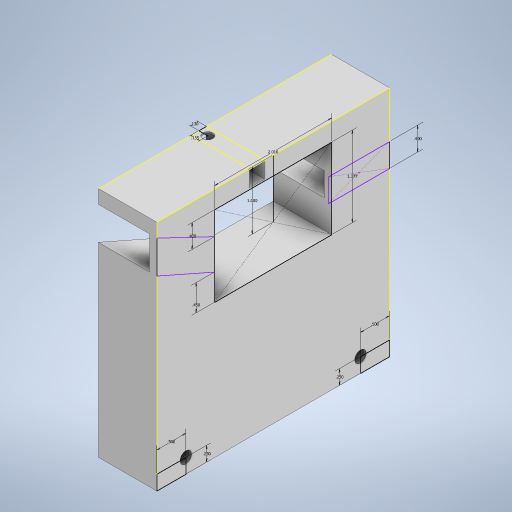
# Autodesk Inventor part: Al thermal core
Saved by Autodesk Inventor 2024.1 (Build 281209000, 209)
## iProperties
Created: 2024-08-21
Part Number: Al thermal core
Material: Generic
Document SubType Name: Modeling
Designer: pab2
Density: 1 g/cm^3
Appearance: Default
Author: pab2
Autodesk Inventor part; units mm, degrees
ref_plane "YZ Plane" through (0, 0, 0) normal (1, 0, 0) x (0, 1, 0)
ref_plane "XZ Plane" through (0, 0, 0) normal (0, 1, 0) x (-1, 0, 0)
ref_plane "XY Plane" through (0, 0, 0) normal (0, 0, 1) x (1, 0, 0)
sketch "Sketch1" plane through (0, 0, 0) normal (1, 0, 0) x (0, 1, 0)
  line L0 (0, 0) -> (101.6, 0)
  line L1 (101.6, 0) -> (101.6, -101.6)
  line L2 (101.6, -101.6) -> (0, -101.6)
  line L3 (0, -101.6) -> (0, 0)
  dimension "d0" = 101.6
  dimension "d1" = 101.6
  constraints: 8 end point, 2 parallel, 1 horizontal, 1 perpendicular
  measures "d0" distance of L1.end L2.end
  measures "d1" distance of L0.end L1.end
extrude "Extrusion1" add sketch "Sketch1" along normal blind 25.4
sketch "Sketch2" plane through (25.4, 0, 0) normal (1, 0, 0) x (0, 0, -1)
  line L0 (0, 101.6) -> (0, 0) projected
  line L1 (0, 0) -> (12.7, 0)
  line L2 (12.7, 0) -> (12.7, 6.35)
  line L3 (12.7, 6.35) -> (0, 6.35)
  line L4 (0, 6.35) -> (0, 0)
  line L5 (101.6, 0) -> (101.6, 101.6) projected
  line L6 (101.6, 0) -> (88.9, 0)
  line L7 (88.9, 0) -> (88.9, 6.35)
  line L8 (88.9, 6.35) -> (101.6, 6.35)
  line L9 (101.6, 6.35) -> (101.6, 0)
  line L10 (101.6, 101.6) -> (0, 101.6) projected
  line L11 (50.8, 101.6) -> (50.8, 76.2)
  line L12 (25.273, 58.7121) -> (76.327, 58.7121)
  line L13 (76.327, 58.7121) -> (76.327, 93.6879)
  line L14 (76.327, 93.6879) -> (25.273, 93.6879)
  line L15 (25.273, 93.6879) -> (25.273, 58.7121)
  line L16 (25.273, 58.7121) -> (76.327, 93.6879) construction
  line L17 (76.327, 58.7121) -> (25.273, 93.6879) construction
  line L18 (74.9076, 71.12) -> (101.6, 71.12)
  line L19 (101.6, 71.12) -> (101.6, 81.28)
  line L20 (101.6, 81.28) -> (74.9076, 81.28)
  line L21 (74.9076, 81.28) -> (74.9076, 71.12)
  line L22 (74.9076, 71.12) -> (101.6, 81.28) construction
  line L23 (101.6, 71.12) -> (74.9076, 81.28) construction
  line L24 (25.273, 93.6879) -> (25.273, 83.5279)
  line L25 (25.273, 58.7121) -> (25.273, 70.1421)
  line L26 (25.273, 70.1421) -> (0, 81.28)
  line L27 (25.273, 83.5279) -> (0, 95.6039)
  line L28 (0, 81.28) -> (0, 95.6039)
  line L29 (25.273, 83.5279) -> (25.273, 70.1421)
  point P0 (88.2538, 76.2)
  point P1 (76.327, 81.28)
  point P2 (76.327, 71.12)
  dimension "d4" = 12.7
  dimension "d5" = 6.35
  dimension "d6" = 12.7
  dimension "d7" = 6.35
  dimension "d8" = 25.4
  dimension "d9" = 51.054
  dimension "d10" = 34.9758
  dimension "d20" = 10.16
  dimension "d21" = 10.16
  dimension "d22" = 11.43
  constraints: 54 end point, 8 parallel, 5 midpoint, 5 point on line, 4 horizontal, 4 perpendicular, 2 collinear, 1 vertical
  measures "d4" distance of L3.end L2.end
  measures "d5" distance of L2.end L1.end
  measures "d6" distance of L7.end L8.end
  measures "d7" distance of L6.end L7.end
  measures "d8" distance of L11.start L11.end
  measures "d9" distance of L14.end L13.end
  measures "d10" distance of L13.end L12.end
  measures "d20" distance of L19.end L18.end
  measures "d21" distance of L14.end L24.end
  measures "d22" distance of L12.start L25.end
extrude "Extrusion2" cut sketch "Sketch2" against normal blind 25.4 contours L27 L15 L26 L0 | L15 L14 L13 L20 L21 L18 L12 | L5 L18 L13 L20 | L13 L18 L21 L20
hole "Hole1" at (25.4, 6.35, -88.9) at (25.4, 6.35, -12.7) direction (-1, 0, 0) diameter 4.9784 end through all thread size "1/4-20 UNC" class "2B" standard "ANSI Unified Screw Threads"
sketch "Sketch5" plane through (25.4, 0, 0) normal (1, 0, 0) x (0, 0, -1)
  line L0 (0, 101.6) -> (0, 95.6039) projected
  line L1 (25.273, 58.7121) -> (76.327, 58.7121) projected
  line L2 (0, 101.6) -> (25.273, 101.6)
  line L3 (25.273, 101.6) -> (25.273, 58.7121)
  line L4 (25.273, 58.7121) -> (0, 58.7121)
  line L5 (0, 58.7121) -> (0, 101.6)
  line L6 (101.6, 81.28) -> (101.6, 101.6) projected
  line L7 (76.327, 58.7121) -> (101.6, 58.7121)
  line L8 (101.6, 58.7121) -> (101.6, 101.6)
  line L9 (101.6, 101.6) -> (76.327, 101.6)
  line L10 (76.327, 101.6) -> (76.327, 58.7121)
  point P0 (0, 0)
  constraints: 16 end point, 4 parallel, 2 horizontal, 2 perpendicular
extrude "Extrusion4" add sketch "Sketch5" against normal blind 3.175
sketch "Sketch6" plane through (25.4, 0, 0) normal (1, 0, 0) x (0, 0, -1)
  line L0 (76.327, 93.6879) -> (25.273, 93.6879) projected
  line L1 (50.8, 93.6879) -> (43.7642, 93.6879)
  line L2 (43.7642, 93.6879) -> (43.7642, 97.6503)
  line L3 (101.6, 101.6) -> (0, 101.6) projected
  line L4 (40.4622, 100.9523) -> (47.0662, 100.9523)
  line L5 (47.0662, 100.9523) -> (47.0662, 94.3483)
  line L6 (47.0662, 94.3483) -> (40.4622, 94.3483)
  line L7 (40.4622, 94.3483) -> (40.4622, 100.9523)
  line L8 (40.4622, 100.9523) -> (47.0662, 94.3483) construction
  line L9 (47.0662, 100.9523) -> (40.4622, 94.3483) construction
  point P0 (0, 0)
  dimension "d30" = 7.0358
  dimension "d31" = 3.9624
  dimension "d32" = 6.604
  dimension "d33" = 6.604
  constraints: 16 end point, 3 midpoint, 2 parallel, 2 perpendicular, 1 horizontal, 1 point on line
  measures "d30" distance of L1.start L1.end
  measures "d31" distance of L1.end L2.end
  measures "d32" distance of L5.end L6.end
  measures "d33" distance of L4.end L5.end
extrude "Extrusion5" cut sketch "Sketch6" against normal blind 25.4
sketch "Sketch7" plane through (0, 101.6, 0) normal (0, 1, 0) x (1, 0, 0)
  line L0 (25.4, 40.4622) -> (0, 40.4622) projected
  line L1 (25.4, 47.0662) -> (0, 47.0662) projected
  line L2 (0, 47.0662) -> (0, 43.7642)
  line L3 (0, 101.6) -> (0, 0) projected
  line L4 (0, 43.7642) -> (3.94, 43.7642)
  dimension "d36" = 3.302
  dimension "d37" = 3.94
  constraints: 4 end point, 1 perpendicular, 1 point on line
  measures "d36" distance of L1.end L2.end
  measures "d37" distance of L2.end L4.end
hole "Hole2" at (3.94, 101.6, -43.7642) direction (0, -1, 0) diameter 4.318 depth 6.35 tip angle 118 clearance for "Socket Head Cap Screw" size "#6" standard "Ansi Unified Screw Threads"
sketch "Sketch8" plane through (25.4, 94.3483, -40.4622) normal (0, 1, 0) x (1, 0, 0)
  point P0 (-25.4, -40.4622)
  point P1 (-21.46, 3.302)
hole "Hole3" at (3.94, 94.3483, -43.7642) direction (0, -1, 0) diameter 2.6416 depth 10.9728 tip angle 118 thread size "6-32 UNC" class "2B" standard "ANSI Unified Screw Threads"
body "Solid1"
